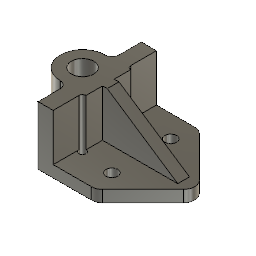
A3 HomeWork 2 (Autodesk Fusion 360 design; units mm, degrees)
Autodesk Fusion 360 part; units mm, degrees
sketch "Sketch1" plane through (0, 0, 0) normal (0, 0, 1) x (1, 0, 0)
  line L0 (0, 88) -> (0, 0)
  line L1 (0, 0) -> (0, 39)
  line L2 (0, 39) -> (0, 49)
  line L3 (0, 39) -> (67, 39)
  line L4 (0, 49) -> (67, 49)
  line L5 (67, 49) -> (67, 39)
  circle A0 centre (67, 44) radius 9.5
  line L6 (67, 44) -> (73.7175, 37.2825)
  circle A1 centre (32.5, 9.5) radius 9.5
  line L7 (39.2175, 2.7825) -> (73.7175, 37.2825)
  line L8 (32.5, 0) -> (0, 0)
  line L9 (0, 44) -> (67, 44)
  line L10 (39.2175, 85.2175) -> (73.7175, 50.7175)
  circle A2 centre (32.5, 78.5) radius 9.5
  line L11 (32.5, 88) -> (0, 88)
  line L12 (67, 44) -> (73.7175, 50.7175)
  line L13 (0, 88) -> (-13, 88)
  line L14 (-13, 88) -> (-13, 0)
  line L15 (0, 4) -> (0, 88)
  line L16 (0, 0) -> (0, 25)
  line L17 (0, 25) -> (3, 25)
  line L18 (3, 25) -> (3, 63)
  line L19 (3, 63) -> (0, 63)
  line L20 (3, 25) -> (3, 39)
  circle A3 centre (-19, 44) radius 9.5
  circle A4 centre (-19, 44) radius 19
  circle A5 centre (31, 19) radius 5
  circle A6 centre (31, 69) radius 5
  circle A7 centre (-19, 19) radius 6
  circle A8 centre (-19, 69) radius 6
  line L21 (-13, 0) -> (0, 0)
  circle A9 centre (3, 22) radius 3
  circle A10 centre (3, 66) radius 3
  dimension "d3" = 39
  dimension "d4" = 10
  dimension "d5" = 19
  dimension "d6" = 19
  dimension "d7" = 45
  dimension "d8" = 45
  dimension "d9" = 13
  dimension "d10" = 25
  dimension "d11" = 3
  dimension "d12" = 38
  dimension "d13" = 14
  dimension "d14" = 19
  dimension "d15" = 19
  dimension "d17" = 38
  dimension "d18" = 10
  dimension "d19" = 31
  dimension "d20" = 25
  dimension "d25" = 12
  dimension "d26" = 88
  dimension "d27" = 44
  dimension "d28" = 6
  constraint vertical L0
  constraint coincident L0.end L1.start
  constraint parallel L0 L2
  constraint coincident A0.centre L6.start
  constraint coincident A0 L6.end
  constraint coincident A1 L7.start
  constraint coincident A1 L8.start
  constraint midpoint L2 L9.start
  constraint perpendicular L5 L9
  constraint symmetric A0.centre L9 L6.start
  constraint symmetric L6.end L9 L10.end
  constraint symmetric A1 L9 A2
  constraint symmetric L7.start L9 L10.start
  constraint symmetric L8.start L9 L11.start
  constraint symmetric L0.end L9 L0.start
  constraint horizontal L13
  constraint vertical L14
  constraint vertical L15
  constraint perpendicular L8 L16
  constraint perpendicular L1 L17
  constraint perpendicular L3 L18
  constraint coincident L15 L19.end
  constraint perpendicular L15 L19
  constraint perpendicular L17 L20
  constraint concentric A3 A4
  constraint symmetric L9 A5 A6
  constraint tangent L14 A7
  constraint tangent A4 A7
  constraint symmetric L9 A7 A8
  constraint perpendicular L1 L21
  constraint coincident L14.end L21.start
  constraint tangent L17 A9
  constraint tangent L16 A9
  constraint symmetric L9 A9 A10
  measures "d3" distance of L0.end L1.end L1.start
  measures "d4" distance of L1.end L2.end
  measures "d5" diameter of A0
  measures "d6" diameter of A1
  measures "d7" angle of L5 L6
  measures "d8" angle of L5 L12
  measures "d9" distance of L0 L14
  measures "d10" distance of L0.end L16.end
  measures "d11" distance of L16.end L17.end
  measures "d12" distance of L17.end L18.end
  measures "d13" distance of L17.end L20.end
  measures "d14" diameter of A3
  measures "d15" distance of L0 A3.centre
  measures "d17" diameter of A4
  measures "d18" diameter of A5
  measures "d19" distance of L1 A5.centre
  measures "d20" distance of L9 A5.centre
  measures "d25" diameter of A7
  measures "d26" distance of L8 L13
  measures "d27" distance of A3.centre L21
  measures "d28" diameter of A9
extrude "Extrude3" add sketch "Sketch1" along normal blind 10 contours L0 L4 A0 L10 A2 L11 L15 L18 A6 A10 | A10 | L4 L5 A0 L12 | A2 A6 | L0 L1 L3 A0 A1 L7 L8 L15 L16 L18 L20 A5 A9 | A0 L6 L12 | L3 L5 A0 L6 | A1 A5 picked at (31.8041, 83.28) picked at (31.8041, 4.72)
extrude "Extrude4" add sketch "Sketch1" along normal blind 50 contours L0 L4 L15 L18 L19 | L0 L2 L13 L14 L15 A4 | L0 L15 L19 A10 | L0 L2 L4 L9 L15 L18 | L0 L2 L3 L9 L15 L18 | L14 A3 A4 | L0 L1 L2 L14 L15 L16 A4 L21 | L4 A0 L9 L18 | L0 L1 L3 L15 L17 L18 L20 | L3 A0 L9 L18 | L14 A4 A8 | L14 A3 A4 | L14 A4 A7 | L4 L5 A0 L9 | L0 L1 L15 L16 L17 A9 | L3 L5 A0 L9
sketch "Sketch2" plane through (0, 39, 0) normal (0, -1, 0) x (1, 0, 0)
  line L0 (3, 10) -> (67, 10)
  line L1 (67, 10) -> (67, 50)
  line L2 (67, 50) -> (3, 50)
  line L3 (3, 50) -> (3, 10)
  line L4 (3, 50) -> (7, 50)
  line L5 (7, 50) -> (67, 10)
  line L6 (7, 50) -> (67, 50)
  line L7 (67, 50) -> (67, 10)
  dimension "d33" = 4
  constraint coincident L2.end L3.start
  constraint perpendicular L3 L4
  constraint coincident L0.end L1.start
  constraint coincident L1.end L2.start
  measures "d33" distance of L2.end L4.end
extrude "Extrude5" cut sketch "Sketch2" against normal blind 10 contours L1 L2 L5 L6 L7
equation "d17 = ( 19 * 2 ) * 1 mm"
